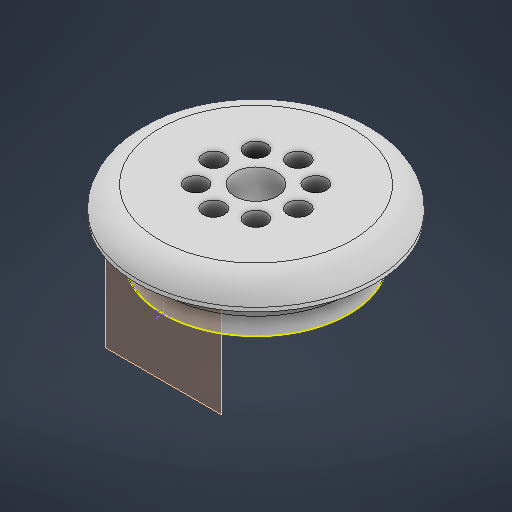
# Autodesk Inventor part: мини катушка 2
Saved by Autodesk Inventor 2025 (Build 290162000, 162)
## iProperties
Created: 2025-02-08
Part Number: мини катушка 2
Material: Типовые
Document SubType Name: Modeling
Designer: Phantom
Density: 1 g/cm^3
Appearance: По умолчанию
Author: Phantom
Autodesk Inventor part; units mm, degrees
ref_plane "YZ Plane" through (0, 0, 0) normal (1, 0, 0) x (0, 1, 0)
ref_plane "XZ Plane" through (0, 0, 0) normal (0, 1, 0) x (-1, 0, 0)
ref_plane "XY Plane" through (0, 0, 0) normal (0, 0, 1) x (1, 0, 0)
sketch "Эскиз1" plane through (0, 0, 0) normal (0, 1, 0) x (-1, 0, 0)
  circle A0 centre (0, 0) radius 17.5
  dimension "d0" = 35
  constraints: 1 centre point, 1 coincident
  measures "d0" diameter of A0
extrude "Выдавливание1" add sketch "Эскиз1" along normal blind 7.5
sketch "Эскиз2" plane through (0, 7.5, 0) normal (0, 1, 0) x (1, 0, 0)
  circle A0 centre (0, 0) radius 22.5
  dimension "d3" = 45
  constraints: 1 centre point, 1 coincident
  measures "d3" diameter of A0
extrude "Выдавливание2" add sketch "Эскиз2" along normal blind 5
fillet "Сопряжение1" radius 4.25 1 edges at (17.5, 7.5, 0)
fillet "Сопряжение2" radius 4.25 1 edges at (-22.5, 12.5, 0)
sketch "Эскиз3" plane through (0, 0, 0) normal (0, -1, 0) x (1, 0, 0)
  line L0 (-24.85, 5.95) -> (-15.15, 5.95)
  line L1 (-15.15, 5.95) -> (-15.15, -5.95)
  line L2 (-15.15, -5.95) -> (-24.85, -5.95)
  line L3 (-24.85, -5.95) -> (-24.85, 5.95)
  line L4 (-4.7, 15.3) -> (-4.7, 25)
  line L5 (-4.7, 25) -> (5, 25)
  line L6 (5, 25) -> (5, 15.3)
  line L7 (5, 15.3) -> (-4.7, 15.3)
  line L8 (5, -15.3) -> (5, -25)
  line L9 (5, -25) -> (-4.7, -25)
  line L10 (-4.7, -25) -> (-4.7, -15.3)
  line L11 (-4.7, -15.3) -> (5, -15.3)
  line L12 (15.15, 5.95) -> (24.85, 5.95)
  line L13 (24.85, 5.95) -> (24.85, -5.95)
  line L14 (24.85, -5.95) -> (15.15, -5.95)
  line L15 (15.15, -5.95) -> (15.15, 5.95)
  circle A0 centre (0, 8) radius 2
  circle A1 centre (-5.6569, -5.6569) radius 2
  circle A2 centre (0, -8) radius 2
  circle A3 centre (0, 0) radius 4
  circle A4 centre (8, 0) radius 2
  circle A5 centre (-8, 0) radius 2
  circle A6 centre (5.6569, -5.6569) radius 2
  circle A7 centre (-5.6569, 5.6569) radius 2
  circle A8 centre (5.6569, 5.6569) radius 2
  circle A9 centre (0, 0) radius 35
  constraints: 32 end point, 10 centre point, 1 coincident
extrude "Выдавливание3" cut sketch "Эскиз3" against normal through all contours A0 | A1 | A2 | A3 | A4 | A5 | A6 | A7 | A8
sketch "Эскиз4" plane through (0, 0, 0) normal (0, -1, 0) x (1, 0, 0)
  circle A0 centre (-8, 0) radius 2 projected
  line L0 (-8, 0) -> (-13.2, 0)
  line L1 (-13.2, 0) -> (-13.2, -2)
  line L2 (-13.2, -2) -> (-15.2, -2)
  line L3 (-15.2, -2) -> (-15.2, 2)
  line L4 (-15.2, 2) -> (-13.2, 2)
  line L5 (-13.2, 2) -> (-13.2, 0)
  line L6 (2, -15.2) -> (-2, -15.2)
  line L7 (2, -13.2) -> (2, -15.2)
  line L8 (-2, -13.2) -> (0, -13.2)
  line L9 (0, -13.2) -> (2, -13.2)
  line L10 (-2, -15.2) -> (-2, -13.2)
  line L11 (15.2, 2) -> (15.2, -2)
  line L12 (13.2, 2) -> (15.2, 2)
  line L13 (13.2, -2) -> (13.2, 0)
  line L14 (13.2, 0) -> (13.2, 2)
  line L15 (15.2, -2) -> (13.2, -2)
  line L16 (-2, 15.2) -> (2, 15.2)
  line L17 (-2, 13.2) -> (-2, 15.2)
  line L18 (2, 13.2) -> (0, 13.2)
  line L19 (0, 13.2) -> (-2, 13.2)
  line L20 (2, 15.2) -> (2, 13.2)
  point P0 (0, 0)
  dimension "d10" = 5.2
  dimension "d11" = 2
  dimension "d12" = 4
  dimension "d15" = 360
  constraints: 42 end point, 5 perpendicular, 4 point on line, 1 horizontal, 41 other
  measures "d10" distance of L0.start L0.end
  measures "d11" distance of L1.end L2.end
  measures "d12" distance of L2.end L3.end
extrude "Выдавливание4" add sketch "Эскиз4" along normal blind 4.5 contours L1 L2 L3 L4 L5 | L6 L10 L8 L9 L7 | L11 L15 L13 L14 L12 | L16 L20 L18 L19 L17
sketch "Эскиз6" plane through (0, 0, 0) normal (0, -1, 0) x (1, 0, 0)
  circle A0 centre (0, 0) radius 17.5 projected
  point P0 (0, 17.5)
  constraints: 1 vertical alignment, 1 other
ref_plane "РабПлоскость1" through (0, 0, 17.5) normal (0, 0, 1) x (1, 0, 0)
sketch "Эскиз8" plane through (0, -4.5, 0) normal (0, -1, 0) x (1, 0, 0)
  line L0 (13.2, 2) -> (13.2, -2) projected
  line L1 (13.2, -2) -> (15.2, -2) projected
  line L2 (15.2, -2) -> (15.2, 2) projected
  line L3 (15.2, 2) -> (13.2, 2) projected
  line L4 (13.05, -2.15) -> (15.35, -2.15)
  line L5 (15.35, -2.15) -> (15.35, 2.15)
  line L6 (15.35, 2.15) -> (13.05, 2.15)
  line L7 (13.05, 2.15) -> (13.05, -2.15)
  line L8 (13.05, -2.15) -> (15.35, 2.15) construction
  line L9 (15.35, -2.15) -> (13.05, 2.15) construction
  line L10 (-2.15, 15.35) -> (-2.15, 13.05)
  line L11 (2.15, 15.35) -> (-2.15, 15.35)
  line L12 (2.15, 13.05) -> (2.15, 15.35)
  line L13 (-2.15, 13.05) -> (2.15, 13.05)
  line L14 (-15.35, -2.15) -> (-13.05, -2.15)
  line L15 (-15.35, 2.15) -> (-15.35, -2.15)
  line L16 (-13.05, 2.15) -> (-15.35, 2.15)
  line L17 (-13.05, -2.15) -> (-13.05, 2.15)
  line L18 (2.15, -15.35) -> (2.15, -13.05)
  line L19 (-2.15, -15.35) -> (2.15, -15.35)
  line L20 (-2.15, -13.05) -> (-2.15, -15.35)
  line L21 (2.15, -13.05) -> (-2.15, -13.05)
  point P0 (0, 0)
  point P1 (14.2, 0)
  dimension "d24" = 2.3
  dimension "d25" = 4.3
  dimension "d28" = 360
  constraints: 36 end point, 2 midpoint, 2 parallel, 1 horizontal, 1 perpendicular, 33 other
  measures "d24" distance of L4.start L4.end
  measures "d25" distance of L5.end L4.end
extrude "Выдавливание6" cut sketch "Эскиз8" against normal blind 9.3 contours L3 L2 L1 L0 | L7 L6 L5 L4 | L11 L12 L13 L10 | L15 L16 L17 L14 | L19 L20 L21 L18
